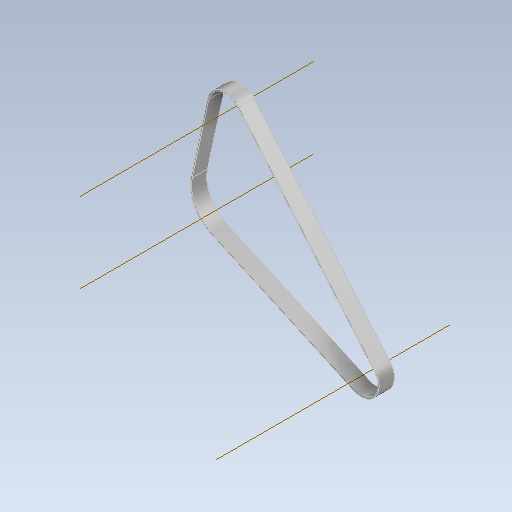
# Autodesk Inventor part: Зубчатый ремень
Saved by Autodesk Inventor 2021 (Build 250183000, 183)
## iProperties
Created: 2021-06-15
Part Number: Зубчатый ремень
Material: Rubber
Document SubType Name: Modeling
Designer: panda
Density: 1 g/cm^3
Appearance: Rubber - Black - Version 1.1
CustomPartVersion: 1
Author: panda
Autodesk Inventor part; units mm, degrees
sketch "Эскизная траектория" plane through (0, 0, 0) normal (0, 0, 1) x (1, 0, 0)
  arc A0 (-41.4791, 9.0112) -> (-17.4646, -38.6872) centre (0, 0) ccw
  arc A1 (16.1709, 113.7164) -> (-20.7395, 104.4767) centre (0, 99.9711) ccw
  arc A2 (161.2677, -119.3725) -> (186.1709, -86.2836) centre (170, -100.0289) ccw
  line L0 (161.2677, -119.3725) -> (-17.4646, -38.6872)
  line L1 (-41.4791, 9.0112) -> (-20.7395, 104.4767)
  line L2 (16.1709, 113.7164) -> (186.1709, -86.2836)
  constraints: 6 end point, 6 point on circle, 3 centre point
ref_plane "Плоскость сечения" through (-17.4646, -38.6872, 0) normal (0.9114, -0.4114, 0) x (0, 0, 1)
ref_plane "РабПлоскость2" through (0, 0, 0) normal (-1, 0, 0) x (0, 0, 1)
ref_plane "РабПлоскость3" through (0, 99.9711, 0) normal (-0.5384, -0.8427, 0) x (0, 0, 1)
ref_plane "РабПлоскость4" through (170, -100.0289, 0) normal (-0.5475, 0.8368, 0) x (0, 0, 1)
sketch "Сечение" plane through (-17.4646, -38.6872, 0) normal (0.9114, -0.4114, 0) x (0, 0, 1)
  line L0 (-9.525, 1.27) -> (9.525, 1.27)
  line L1 (9.525, 1.27) -> (9.525, -0.381)
  line L2 (9.525, -0.381) -> (-9.525, -0.381)
  line L3 (-9.525, -0.381) -> (-9.525, 1.27)
  line L4 (-9.525, 0) -> (9.525, 0) construction
  point P0 (0, 0)
  point P1 (0, 0)
  dimension "d0" = 19.05
  dimension "d4" = 0.381
  dimension "d5" = 1.27
  constraints: 10 end point, 2 parallel, 2 point on line, 1 coincident, 1 horizontal, 1 midpoint, 1 perpendicular, 1 other
  measures "d0" distance between parallel lines of L1 L3
  measures "d4" distance between parallel lines of L2 L4
  measures "d5" distance between parallel lines of L4 L0
sweep "Ремень" add profiles "Сечение" path "Эскизная траектория"
equation "\"d0\" = da_B"
equation "\"d4\" = da_a"
equation "\"d5\" = da_a2"
equation "\"da_B\" = 19.05"
equation "\"da_pb\" = 9.525"
equation "\"da_L\" = 718.50884"
equation "\"da_a\" = 0.381"
equation "\"da_S\" = 4.6482"
equation "\"da_Beta\" = 20deg"
equation "\"da_Ht\" = 1.905"
equation "\"da_H\" = 3.556"
equation "\"da_a2\" = 1.27"
body "Solid1"
